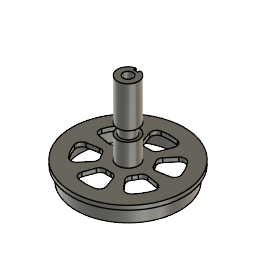
Front Reel Shaft (Autodesk Fusion 360 design; units mm, degrees)
Autodesk Fusion 360 part; units mm, degrees
sketch "Sketch1" plane through (0, 0, 0) normal (0, 0, 1) x (1, 0, 0)
  circle A0 centre (0, 0) radius 33.9
  circle A1 centre (0, 0) radius 36.9
  circle A2 centre (0, 0) radius 39.9
  circle A3 centre (0, 0) radius 7.5
  circle A4 centre (0, 0) radius 14
  line L0 (0, 0) -> (4.7883, -13.1557)
  line L1 (0, 0) -> (-4.7883, -13.1557)
  line L2 (0, -60) -> (0, 60)
  line L3 (4.7883, -13.1557) -> (10.2606, -28.1908)
  line L4 (-4.7883, -13.1557) -> (-10.2606, -28.1908)
  arc A5 (10.2606, -28.1908) -> (-10.2606, -28.1908) centre (0, 0) ccw
  arc A6 (-10.2606, -28.1908) -> (0, -30) centre (0, 0) ccw
  arc A7 (0, -30) -> (10.2606, -28.1908) centre (0, 0) ccw
  line L5 (13.7873, -2.4311) -> (29.5442, -5.2094)
  line L6 (8.999, -10.7246) -> (19.2836, -22.9813)
  line L7 (8.999, 10.7246) -> (19.2836, 22.9813)
  line L8 (13.7873, 2.4311) -> (29.5442, 5.2094)
  line L9 (-4.7883, 13.1557) -> (-10.2606, 28.1908)
  line L10 (4.7883, 13.1557) -> (10.2606, 28.1908)
  line L11 (-13.7873, 2.4311) -> (-29.5442, 5.2094)
  line L12 (-8.999, 10.7246) -> (-19.2836, 22.9813)
  line L13 (-8.999, -10.7246) -> (-19.2836, -22.9813)
  line L14 (-13.7873, -2.4311) -> (-29.5442, -5.2094)
  circle A8 centre (0, 0) radius 3.5
  line L15 (-1.5, 7.3485) -> (-1.5, 5.5)
  line L16 (-1.5, 5.5) -> (1.5, 5.5)
  line L17 (1.5, 5.5) -> (1.5, 7.3485)
  circle A9 centre (0, 0) radius 5.5
  point P0 (0, 7.5)
  dimension "d1" = 67.8
  dimension "d2" = 3
  dimension "d3" = 3
  dimension "d4" = 15
  dimension "d11" = 28
  dimension "d12" = 60
  dimension "d13" = 40
  dimension "d15" = 20
  dimension "d17" = 360
  dimension "d22" = -4
  dimension "d34" = 3
  dimension "d35" = 2
  dimension "d43" = -2
  constraint coincident A0.centre A1.centre
  constraint concentric A0 A3
  constraint concentric A0 A5
  constraint concentric A0 A4
  constraint vertical L2
  constraint coincident A4 L0.end
  constraint coincident A4 L1.end
  constraint coincident L2 A6.end
  constraint concentric A5 A6
  constraint concentric A5 A7
  constraint coincident A3 L15.start
  constraint vertical L15
  constraint perpendicular L2 L16
  constraint coincident A3 L17.end
  constraint perpendicular L16 L17
  constraint symmetric L2 L15 L17
  constraint coincident A3 P0
  constraint coincident L2 P0
  constraint coincident A0.centre L2
  measures "d1" diameter of A0
  measures "d4" diameter of A3
  measures "d11" diameter of A4
  measures "d12" diameter of A5
  measures "d13" angle of L0 L1
  measures "d15" angle of L1 L2
  measures "d34" distance of L15.end L16.end
  measures "d35" distance of L16 P0
extrude "Extrude1" add sketch "Sketch1" against normal blind 10 contours A0 A1 L2 | A0 A1 L2
extrude "Extrude2" add sketch "Sketch1" along normal blind 3
extrude "Extrude3" add sketch "Sketch1" along normal blind 55 contours A3 L2 L15 L16 | A3 L2 L16 L17 | A3 L0 L2 A9 | A3 L1 L2 A9 | A3 L0 L16 L17 A9 | A3 L1 L15 L16 A9 | L0 L2 A8 A9 | L1 L2 A8 A9 | L1 L2 A8 A9 | L0 L2 A8 A9 | L0 L2 A8 | L1 L2 A8 | L1 L2 A8 | L0 L2 A8
extrude "Extrude4" cut sketch "Sketch1" along normal blind 3 contours A4 L2 A5 L10 | A4 L2 A5 L9 | A4 L2 L4 A6 | A4 L2 L3 A7 | A4 A5 L7 L8 | A4 A5 L11 L12 | A4 A5 L13 L14 | A4 A5 L5 L6
fillet "Fillet1" radius 4 24 edges at (-19.2836, 22.9813, 1.5) (-29.5442, 5.2094, 1.5) (-13.7873, 2.4311, 1.5) (-8.999, 10.7246, 1.5) (-13.7873, -2.4311, 1.5) (-29.5442, -5.2094, 1.5) (-19.2836, -22.9813, 1.5) (-8.999, -10.7246, 1.5) (-4.7883, -13.1557, 1.5) (-10.2606, -28.1908, 1.5) (10.2606, -28.1908, 1.5) (4.7883, -13.1557, 1.5) (8.999, -10.7246, 1.5) (19.2836, -22.9813, 1.5) (29.5442, -5.2094, 1.5) (13.7873, -2.4311, 1.5) (29.5442, 5.2094, 1.5) (19.2836, 22.9813, 1.5) (13.7873, 2.4311, 1.5) (8.999, 10.7246, 1.5) (4.7883, 13.1557, 1.5) (10.2606, 28.1908, 1.5) (-4.7883, 13.1557, 1.5) (-10.2606, 28.1908, 1.5)
extrude "Extrude5" cut sketch "Sketch1" against normal up to surface (52 mm away) from surface at 55 contours L0 L2 A8 | L1 L2 A8 | L1 L2 A8 | L0 L2 A8
extrude "Extrude8" cut sketch "Sketch1" against normal blind 25 from surface at 55 contours A3 L2 L15 L16 | A3 L2 L16 L17
extrude "Extrude9" cut sketch "Sketch1" along normal blind 7 from surface at 19 contours A3 L2 L15 L16 | A3 L2 L16 L17 | A3 L0 L2 A9 | A3 L1 L2 A9 | A3 L0 L16 L17 A9 | A3 L1 L15 L16 A9
